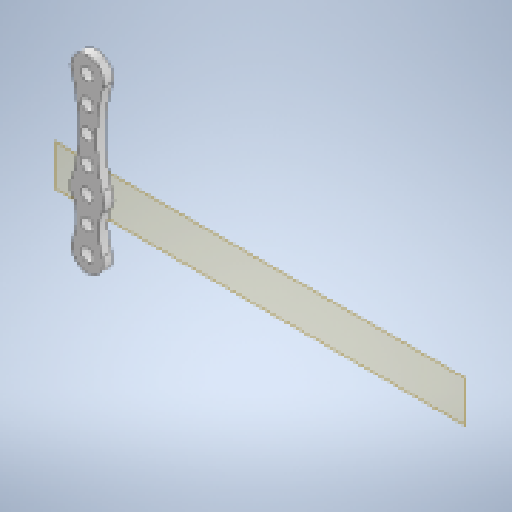
# Autodesk Inventor part: see-saw-arm
Saved by Autodesk Inventor 2024.1 (Build 281209000, 209)
## iProperties
Created: 2025-06-10
Part Number: see-saw-arm
Material: Generic
Document SubType Name: Modeling
Designer: iwheard
Density: 1 g/cm^3
Appearance: Default
Author: iwheard
Autodesk Inventor part; units mm, degrees
ref_plane "YZ Plane" through (0, 0, 0) normal (1, 0, 0) x (0, 1, 0)
ref_plane "XZ Plane" through (0, 0, 0) normal (0, 1, 0) x (-1, 0, 0)
ref_plane "XY Plane" through (0, 0, 0) normal (0, 0, 1) x (1, 0, 0)
ref_plane "Work Plane1" through (0, 0, 0) normal (0, 0, 1) x (1, 0, 0)
sketch "Sketch1" plane through (0, 0, 0) normal (0, 0, 1) x (1, 0, 0)
  circle A0 centre (-44, 0) radius 1.6 projected
  circle A1 centre (-44, 0) radius 4.6
  line L0 (-48.6, 50) -> (-48.6, -25) construction
  circle A2 centre (-44, 0) radius 1.6
  circle A3 centre (-44, -7) radius 1.6
  circle A4 centre (-44, -7) radius 4.6
  circle A5 centre (-44, 7) radius 1.6
  circle A6 centre (-44, 7) radius 4.6
  circle A7 centre (-44, 0) radius 1.6
  circle A8 centre (-44, 0) radius 4.6
  circle A9 centre (-44, 14) radius 1.6
  circle A10 centre (-44, 14) radius 4.6
  circle A11 centre (-44, 7) radius 1.6
  circle A12 centre (-44, 7) radius 4.6
  circle A13 centre (-44, 21) radius 1.6
  circle A14 centre (-44, 21) radius 4.6
  circle A15 centre (-44, 14) radius 1.6
  circle A16 centre (-44, 14) radius 4.6
  circle A17 centre (-44, -14) radius 1.6
  circle A18 centre (-44, -14) radius 4.6
  circle A19 centre (-44, -7) radius 1.6
  circle A20 centre (-44, -7) radius 4.6
  circle A21 centre (-44, 0) radius 1.6
  circle A22 centre (-44, 0) radius 4.6
  circle A23 centre (-44, 7) radius 1.6
  circle A24 centre (-44, 7) radius 4.6
  circle A25 centre (-44, 28) radius 1.6
  circle A26 centre (-44, 28) radius 4.6
  circle A27 centre (-44, 21) radius 1.6
  circle A28 centre (-44, 21) radius 4.6
  circle A29 centre (-44, 14) radius 1.6
  circle A30 centre (-44, 14) radius 4.6
  arc A31 (-39.4, 0) -> (-39.4, -14) centre (-24.8875, -7) ccw
  arc A32 (-39.4, 28) -> (-39.4, 0) centre (4.0455, 14) ccw
  arc A33 (-48.6, -14) -> (-48.6, 0) centre (-63.1125, -7) ccw
  arc A34 (-48.6, 0) -> (-48.6, 28) centre (-92.0455, 14) ccw
  circle A35 centre (-44, -14) radius 4.2416
  circle A36 centre (-44, 28) radius 4.3982
  point P0 (0, 0)
  point P1 (-41.6, 14)
  point P2 (-41, -7)
  point P3 (-47, -7)
  point P4 (-46.4, 14)
  point P5 (-40.4881, -11.029)
  point P6 (-40.4881, -2.971)
  point P7 (-47.5119, -2.971)
  point P8 (-47.5119, -11.029)
  point P9 (-40.12, 2.471)
  point P10 (-40.12, 25.529)
  point P11 (-47.88, 25.529)
  point P12 (-47.88, 2.471)
  point P13 (-39.7774, 26.7696)
  point P14 (-48.2226, 26.7696)
  point P15 (-47.9828, -12.5413)
  point P16 (-40.0172, -12.5413)
  dimension "d0" = 3
  dimension "d1" = 9.2
  dimension "d8" = 7
  dimension "d11" = 7
  dimension "d18" = 2.4
  dimension "d19" = 3
  dimension "d20" = 3
  dimension "d21" = 2.4
  constraints: 36 centre point, 18 point on circle, 17 coincident, 3 point on line, 2 end point, 2 tangent, 2 vertical, 1 concentric, 56 other
  measures "d0" radial gap between concentric circles of A1 A0
  measures "d1" diameter of A1
  measures "d8" distance of A2.centre A3.centre
  measures "d11" distance of A2.centre A5.centre
  measures "d18" distance of point (-41.6, 14) A9.centre
  measures "d19" distance of A3.centre point (-41, -7)
  measures "d20" distance of point (-47, -7) A3.centre
  measures "d21" distance of A9.centre point (-46.4, 14)
extrude "Extrusion1" add sketch "Sketch1" along normal blind 2.5 contours A32 A1 | A1 A31 | A31 A1 A4 A33 A34 A6 A32 | A1 A6 A32 | A31 A4 A1 | A6 A1 | A1 A6 A34 A10 A32 | A4 A31 A18 A33 A1 | A1 A4 | A1 A34 A6 | A10 A34 A6 A32 | A4 A33 A1 | A31 A18 A4 | A34 A1 | A6 A34 A14 A32 | A1 A33 | A18 A31 A35 A4 | A4 A35 A18 | A14 A34 A10 A32 | A4 A18 A33 | A35 A4 | A4 A35 | A4 A35 A33 A18 | A10 A34 A14 A26 A32 | A34 A26 A14 | A14 A26 A32 | A26 A34 A36 A14 | A14 A36 A26 | A14 A36 A32 A26 | A36 A14 | A14 A36
equation "\"d20\" = d19"
equation "\"d21\" = d18"
